Autodesk Fusion 360 part; units mm, degrees
note: some values were not read from the file. Chosen so that the rebuilt part matches the saved one: which face or edge a step refers to. Set by a fixed rule: which sketch regions a step uses.
(part 2 of 7)
  arc A150 (-15.4464, 34.8123) -> (-14.944, 34.6491) centre (-15.1024, 35.0164) ccw
  spline S149 degree 3 poles (-19.866, 37.3046) (-19.823, 35.7503) (-19.6037, 34.6096) (-19.3931, 33.8552) knots 0 0 0 0 1 1 1 1
  arc A151 (-20.7021, 31.9674) -> (-20.1803, 31.8848) centre (-20.3942, 32.2228) ccw
  spline S150 degree 3 poles (-10.2263, 37.6523) (-10.6107, 38.3346) (-11.2623, 39.2962) (-12.331, 40.4257) knots 0 0 0 0 1 1 1 1
  spline S151 degree 3 poles (-13.8582, 36.4722) (-13.808, 36.0399) (-13.7432, 35.732) (-13.6938, 35.5383) knots 0 0 0 0 1 1 1 1
  arc A152 (-8.2763, 36.8156) -> (-9.3397, 36.5603) centre (0, 0) ccw
  spline S152 degree 3 poles (-1.9094, 38.9695) (-1.9952, 38.5429) (-2.0288, 38.23) (-2.0416, 38.0306) knots 0 0 0 0 1 1 1 1
  spline S153 degree 3 poles (-20.7021, 31.9674) (-20.8297, 32.1213) (-21.0408, 32.3546) (-21.3609, 32.6493) knots 0 0 0 0 1 1 1 1
  arc A153 (-19.2479, 32.4562) -> (-20.1803, 31.8848) centre (0, 0) ccw
  spline S154 degree 3 poles (-7.9821, 38.191) (-8.0001, 37.7562) (-7.9843, 37.442) (-7.9658, 37.243) knots 0 0 0 0 1 1 1 1
  arc A154 (-9.8104, 36.8001) -> (-9.3397, 36.5603) centre (-9.4387, 36.9478) ccw
  arc A155 (-13.9336, 35.0676) -> (-14.944, 34.6491) centre (0, 0) ccw
  spline S155 degree 3 poles (-13.7857, 39.953) (-13.9863, 38.4112) (-13.9482, 37.2502) (-13.8582, 36.4722) knots 0 0 0 0 1 1 1 1
  arc A156 (-18.5031, 37.999) -> (-19.866, 37.3046) centre (0, 0) ccw
  arc A157 (-19.2479, 32.4562) -> (-19.0846, 32.9586) centre (-19.4519, 32.8002) ccw
  arc A158 (-24.0882, 29.0455) -> (-24.0055, 29.5673) centre (-24.3435, 29.3534) ccw
  spline S156 degree 3 poles (-25.4571, 33.7376) (-25.1715, 32.2092) (-24.7765, 31.1168) (-24.4505, 30.4047) knots 0 0 0 0 1 1 1 1
  arc A159 (-24.2197, 34.6367) -> (-25.4571, 33.7376) centre (0, 0) ccw
  arc A160 (-24.0882, 29.0455) -> (-24.9197, 28.3353) centre (0, 0) ccw
  spline S157 degree 3 poles (-15.9905, 35.5889) (-16.477, 36.2028) (-17.271, 37.0506) (-18.5031, 37.999) knots 0 0 0 0 1 1 1 1
  spline S158 degree 3 poles (-19.3931, 33.8552) (-19.2759, 33.4362) (-19.1638, 33.1422) (-19.0846, 32.9586) knots 0 0 0 0 1 1 1 1
  spline S159 degree 3 poles (-21.3609, 32.6493) (-21.9375, 33.1795) (-22.8543, 33.8927) (-24.2197, 34.6367) knots 0 0 0 0 1 1 1 1
extrude "Extrude1'" add sketch "sketch 26269" along normal blind 8 separate body makes body 2 in component "Spur Gear (40 teeth)"
sketch "Sketch1 (2)" plane through (0, 0, 0) normal (0, 1, 0) x (1, 0, 0) in component "Spur Gear (40 teeth)"
  circle A0 centre (0, 0) radius 40.25 construction
sketch "sketch 33723" plane through (0, 0, 0) normal (0, 1, 0) x (1, 0, 0)
  arc A0 (-65.084, 44.4151) -> (-65.9408, 43.1328) centre (0, 0) ccw
  arc A1 (-66.3817, 42.9661) -> (-65.9408, 43.1328) centre (-66.2755, 43.3518) ccw
  arc A2 (-65.084, 44.4151) -> (-65.0987, 44.8863) centre (-65.4144, 44.6406) ccw
  arc A3 (-66.0742, 48.9963) -> (-67.0163, 47.6996) centre (0, 0) ccw
  arc A4 (-61.3986, 49.3846) -> (-62.3533, 48.1735) centre (0, 0) ccw
  spline S0 degree 3 poles (-66.9941, 43.1264) (-66.7812, 43.0736) (-66.5772, 43.02) (-66.3817, 42.9661) knots 0 0 0 0 1 1 1 1
  spline S1 degree 3 poles (-65.0987, 44.8863) (-65.2233, 45.0463) (-65.3508, 45.2143) (-65.4811, 45.3907) knots 0 0 0 0 1 1 1 1
  arc A5 (-58.8431, 52.8215) -> (-58.3815, 52.9172) centre (-58.6778, 53.1858) ccw
  arc A6 (-57.3346, 54.0497) -> (-58.3815, 52.9172) centre (0, 0) ccw
  spline S2 degree 3 poles (-62.0263, 54.0294) (-61.0366, 53.717) (-60.1704, 53.3921) (-59.4228, 53.0756) knots 0 0 0 0 1 1 1 1
  spline S3 degree 3 poles (-63.4039, 48.2497) (-63.1959, 48.1804) (-62.9966, 48.111) (-62.806, 48.0419) knots 0 0 0 0 1 1 1 1
  arc A7 (-62.806, 48.0419) -> (-62.3533, 48.1735) centre (-62.6699, 48.418) ccw
  spline S4 degree 3 poles (-61.7179, 50.3883) (-62.1475, 51.0772) (-62.6039, 51.8819) (-63.0673, 52.8106) knots 0 0 0 0 1 1 1 1
  spline S5 degree 3 poles (-61.3763, 49.8555) (-61.4879, 50.0247) (-61.6019, 50.2023) (-61.7179, 50.3883) knots 0 0 0 0 1 1 1 1
  spline S6 degree 3 poles (-65.4811, 45.3907) (-65.9633, 46.0437) (-66.4815, 46.8101) (-67.0163, 47.6996) knots 0 0 0 0 1 1 1 1
  arc A8 (-57.3346, 54.0497) -> (-57.2755, 54.5174) centre (-57.6257, 54.324) ccw
  arc A9 (-61.3986, 49.3846) -> (-61.3763, 49.8555) centre (-61.7102, 49.6353) ccw
  spline S7 degree 3 poles (-66.0742, 48.9963) (-65.063, 48.7626) (-64.174, 48.5066) (-63.4039, 48.2497) knots 0 0 0 0 1 1 1 1
  arc A10 (-62.0263, 54.0294) -> (-63.0673, 52.8106) centre (0, 0) ccw
  spline S8 degree 3 poles (-52.8106, 63.0673) (-51.8819, 62.6039) (-51.0772, 62.1475) (-50.3883, 61.7179) knots 0 0 0 0 1 1 1 1
  spline S9 degree 3 poles (-59.4228, 53.0756) (-59.2209, 52.9901) (-59.0277, 52.9053) (-58.8431, 52.8215) knots 0 0 0 0 1 1 1 1
  spline S10 degree 3 poles (-57.2755, 54.5174) (-57.3735, 54.6948) (-57.4732, 54.8807) (-57.5742, 55.0753) knots 0 0 0 0 1 1 1 1
  arc A11 (-57.596, 58.7294) -> (-58.7294, 57.596) centre (0, 0) ccw
  spline S11 degree 3 poles (-57.5742, 55.0753) (-57.9484, 55.7958) (-58.3403, 56.6338) (-58.7294, 57.596) knots 0 0 0 0 1 1 1 1
  spline S12 degree 3 poles (-57.596, 58.7294) (-56.6338, 58.3403) (-55.7958, 57.9484) (-55.0753, 57.5742) knots 0 0 0 0 1 1 1 1
  spline S13 degree 3 poles (-55.0753, 57.5742) (-54.8807, 57.4732) (-54.6948, 57.3735) (-54.5174, 57.2755) knots 0 0 0 0 1 1 1 1
  arc A12 (-52.9172, 58.3815) -> (-52.8215, 58.8431) centre (-53.1858, 58.6778) ccw
  arc A13 (-54.5174, 57.2755) -> (-54.0497, 57.3346) centre (-54.324, 57.6257) ccw
  arc A14 (-52.9172, 58.3815) -> (-54.0497, 57.3346) centre (0, 0) ccw
  spline S14 degree 3 poles (-50.3883, 61.7179) (-50.2023, 61.6019) (-50.0247, 61.4879) (-49.8555, 61.3763) knots 0 0 0 0 1 1 1 1
  spline S15 degree 3 poles (-52.8215, 58.8431) (-52.9053, 59.0277) (-52.9901, 59.2209) (-53.0756, 59.4228) knots 0 0 0 0 1 1 1 1
  spline S16 degree 3 poles (-48.0419, 62.806) (-48.111, 62.9966) (-48.1804, 63.1959) (-48.2497, 63.4039) knots 0 0 0 0 1 1 1 1
  arc A15 (-48.1735, 62.3533) -> (-49.3846, 61.3986) centre (0, 0) ccw
  arc A16 (-52.8106, 63.0673) -> (-54.0294, 62.0263) centre (0, 0) ccw
  spline S17 degree 3 poles (-53.0756, 59.4228) (-53.3921, 60.1704) (-53.717, 61.0366) (-54.0294, 62.0263) knots 0 0 0 0 1 1 1 1
  arc A17 (-49.8555, 61.3763) -> (-49.3846, 61.3986) centre (-49.6353, 61.7102) ccw
  spline S18 degree 3 poles (-47.6996, 67.0163) (-46.8101, 66.4815) (-46.0437, 65.9633) (-45.3907, 65.4811) knots 0 0 0 0 1 1 1 1
  spline S19 degree 3 poles (-48.2497, 63.4039) (-48.5066, 64.174) (-48.7626, 65.063) (-48.9963, 66.0742) knots 0 0 0 0 1 1 1 1
  arc A18 (-48.1735, 62.3533) -> (-48.0419, 62.806) centre (-48.418, 62.6699) ccw
  spline S20 degree 3 poles (-45.3907, 65.4811) (-45.2143, 65.3508) (-45.0463, 65.2233) (-44.8863, 65.0987) knots 0 0 0 0 1 1 1 1
  arc A19 (-43.1328, 65.9408) -> (-44.4151, 65.084) centre (0, 0) ccw
  arc A20 (-43.1328, 65.9408) -> (-42.9661, 66.3817) centre (-43.3518, 66.2755) ccw
  spline S21 degree 3 poles (-42.9661, 66.3817) (-43.02, 66.5772) (-43.0736, 66.7812) (-43.1264, 66.9941) knots 0 0 0 0 1 1 1 1
  arc A21 (-44.8863, 65.0987) -> (-44.4151, 65.084) centre (-44.6406, 65.4144) ccw
  spline S22 degree 3 poles (-42.2945, 70.5522) (-41.4498, 69.9493) (-40.7264, 69.3726) (-40.1132, 68.8406) knots 0 0 0 0 1 1 1 1
  arc A22 (-39.6403, 68.4198) -> (-39.1718, 68.3681) centre (-39.3706, 68.7152) ccw
  arc A23 (-47.6996, 67.0163) -> (-48.9963, 66.0742) centre (0, 0) ccw
  arc A24 (-42.2945, 70.5522) -> (-43.6612, 69.7147) centre (0, 0) ccw
  spline S23 degree 3 poles (-40.1132, 68.8406) (-39.9475, 68.6969) (-39.79, 68.5565) (-39.6403, 68.4198) knots 0 0 0 0 1 1 1 1
  spline S24 degree 3 poles (-37.7371, 70.1712) (-37.8704, 70.972) (-37.9841, 71.8901) (-38.0568, 72.9254) knots 0 0 0 0 1 1 1 1
  spline S25 degree 3 poles (-37.6254, 69.5482) (-37.6638, 69.7473) (-37.7012, 69.9549) (-37.7371, 70.1712) knots 0 0 0 0 1 1 1 1
  spline S26 degree 3 poles (-43.1264, 66.9941) (-43.322, 67.7819) (-43.5075, 68.6883) (-43.6612, 69.7147) knots 0 0 0 0 1 1 1 1
  arc A25 (-37.8262, 69.1217) -> (-39.1718, 68.3681) centre (0, 0) ccw
  spline S27 degree 3 poles (-30.737, 76.2999) (-29.997, 75.5723) (-29.3727, 74.8895) (-28.8503, 74.2681) knots 0 0 0 0 1 1 1 1
  arc A26 (-34.15, 71.319) -> (-33.6869, 71.2307) centre (-33.8579, 71.5923) ccw
  arc A27 (-26.5475, 74.188) -> (-27.9944, 73.6542) centre (0, 0) ccw
  arc A28 (-26.5475, 74.188) -> (-26.2825, 74.5778) centre (-26.6822, 74.5646) ccw
  spline S28 degree 3 poles (-34.5883, 71.7756) (-34.4345, 71.6193) (-34.2885, 71.4671) (-34.15, 71.319) knots 0 0 0 0 1 1 1 1
  arc A29 (-32.2864, 71.8764) -> (-32.0528, 72.2858) centre (-32.4503, 72.2413) ccw
  arc A30 (-36.6287, 73.6531) -> (-38.0568, 72.9254) centre (0, 0) ccw
  spline S29 degree 3 poles (-32.0528, 72.2858) (-32.0754, 72.4873) (-32.0964, 72.6972) (-32.1152, 72.9157) knots 0 0 0 0 1 1 1 1
  arc A31 (-30.737, 76.2999) -> (-32.2178, 75.6865) centre (0, 0) ccw
  spline S30 degree 3 poles (-26.2825, 74.5778) (-26.2892, 74.7805) (-26.2937, 74.9914) (-26.2953, 75.2107) knots 0 0 0 0 1 1 1 1
  arc A32 (-32.2864, 71.8764) -> (-33.6869, 71.2307) centre (0, 0) ccw
  spline S31 degree 3 poles (-28.8503, 74.2681) (-28.7092, 74.1003) (-28.5755, 73.937) (-28.4491, 73.7785) knots 0 0 0 0 1 1 1 1
  arc A33 (-37.8262, 69.1217) -> (-37.6254, 69.5482) centre (-38.0182, 69.4726) ccw
  spline S32 degree 3 poles (-36.6287, 73.6531) (-35.8338, 72.9858) (-35.1579, 72.3541) (-34.5883, 71.7756) knots 0 0 0 0 1 1 1 1
  spline S33 degree 3 poles (-32.1152, 72.9157) (-32.1852, 73.7245) (-32.2266, 74.6487) (-32.2178, 75.6865) knots 0 0 0 0 1 1 1 1
  arc A34 (-28.4491, 73.7785) -> (-27.9944, 73.6542) centre (-28.1365, 74.0281) ccw
  spline S34 degree 3 poles (-26.2953, 75.2107) (-26.3016, 76.0225) (-26.2704, 76.9471) (-26.1802, 77.981) knots 0 0 0 0 1 1 1 1
  arc A35 (-24.6558, 78.4763) -> (-26.1802, 77.981) centre (0, 0) ccw
  arc A36 (-20.6449, 76.0422) -> (-22.1292, 75.6235) centre (0, 0) ccw
  arc A37 (-20.6449, 76.0422) -> (-20.3501, 76.41) centre (-20.7497, 76.4282) ccw
  spline S35 degree 3 poles (-24.6558, 78.4763) (-23.9752, 77.6928) (-23.4064, 76.9632) (-22.9343, 76.3027) knots 0 0 0 0 1 1 1 1
  spline S36 degree 3 poles (-22.9343, 76.3027) (-22.8068, 76.1243) (-22.6864, 75.9511) (-22.5728, 75.7832) knots 0 0 0 0 1 1 1 1
  arc A38 (-22.5728, 75.7832) -> (-22.1292, 75.6235) centre (-22.2416, 76.0074) ccw
  spline S37 degree 3 poles (-20.3133, 77.0419) (-20.2559, 77.8517) (-20.1522, 78.771) (-19.9812, 79.7947) knots 0 0 0 0 1 1 1 1
  arc A39 (-18.4227, 80.1689) -> (-19.9812, 79.7947) centre (0, 0) ccw
  arc A40 (-14.6151, 77.4275) -> (-14.2923, 77.7712) centre (-14.6893, 77.8206) ccw
  spline S38 degree 3 poles (-20.3501, 76.41) (-20.341, 76.6126) (-20.3288, 76.8232) (-20.3133, 77.0419) knots 0 0 0 0 1 1 1 1
  spline S39 degree 3 poles (-18.4227, 80.1689) (-17.8055, 79.3344) (-17.2958, 78.5624) (-16.877, 77.8669) knots 0 0 0 0 1 1 1 1
  spline S40 degree 3 poles (-14.2061, 78.3982) (-14.0853, 79.201) (-13.9098, 80.1093) (-13.659, 81.1164) knots 0 0 0 0 1 1 1 1
  arc A41 (-16.5573, 77.3206) -> (-16.1277, 77.1267) centre (-16.2095, 77.5182) ccw
  arc A42 (-14.6151, 77.4275) -> (-16.1277, 77.1267) centre (0, 0) ccw
  arc A43 (-12.0759, 81.3672) -> (-13.659, 81.1164) centre (0, 0) ccw
  spline S41 degree 3 poles (-14.2923, 77.7712) (-14.2673, 77.9723) (-14.2387, 78.1814) (-14.2061, 78.3982) knots 0 0 0 0 1 1 1 1
  spline S42 degree 3 poles (-16.877, 77.8669) (-16.7639, 77.6791) (-16.6574, 77.4969) (-16.5573, 77.3206) knots 0 0 0 0 1 1 1 1
  spline S43 degree 3 poles (-12.0759, 81.3672) (-11.5261, 80.4868) (-11.0785, 79.6772) (-10.7156, 78.951) knots 0 0 0 0 1 1 1 1
  arc A44 (-5.6547, 82.0638) -> (-7.2526, 81.938) centre (0, 0) ccw
  arc A45 (-10.4398, 78.3813) -> (-10.0267, 78.1543) centre (-10.0776, 78.551) ccw
  spline S44 degree 3 poles (-10.7156, 78.951) (-10.6176, 78.7549) (-10.5258, 78.5649) (-10.4398, 78.3813) knots 0 0 0 0 1 1 1 1
  arc A46 (-8.4951, 78.3355) -> (-10.0267, 78.1543) centre (0, 0) ccw
  arc A47 (-8.4951, 78.3355) -> (-8.1464, 78.6528) centre (-8.5383, 78.7332) ccw
  spline S45 degree 3 poles (-8.0112, 79.2711) (-7.8278, 80.0619) (-7.5816, 80.9537) (-7.2526, 81.938) knots 0 0 0 0 1 1 1 1
  spline S46 degree 3 poles (-8.1464, 78.6528) (-8.1057, 78.8514) (-8.0608, 79.0575) (-8.0112, 79.2711) knots 0 0 0 0 1 1 1 1
  arc A48 (-78.1543, 10.0267) -> (-78.3355, 8.4951) centre (0, 0) ccw
  arc A49 (-77.1267, 16.1277) -> (-77.3206, 16.5573) centre (-77.5182, 16.2095) ccw
  spline S47 degree 3 poles (-77.8669, 16.877) (-78.5624, 17.2958) (-79.3344, 17.8055) (-80.1689, 18.4227) knots 0 0 0 0 1 1 1 1
  arc A50 (-79.7947, 19.9812) -> (-80.1689, 18.4227) centre (0, 0) ccw
  spline S48 degree 3 poles (-81.1164, 13.659) (-80.1093, 13.9098) (-79.201, 14.0853) (-78.3982, 14.2061) knots 0 0 0 0 1 1 1 1
  spline S49 degree 3 poles (-78.3982, 14.2061) (-78.1814, 14.2387) (-77.9723, 14.2673) (-77.7712, 14.2923) knots 0 0 0 0 1 1 1 1
  arc A51 (-75.6235, 22.1292) -> (-76.0422, 20.6449) centre (0, 0) ccw
  arc A52 (-77.1267, 16.1277) -> (-77.4275, 14.6151) centre (0, 0) ccw
  arc A53 (-75.6235, 22.1292) -> (-75.7832, 22.5728) centre (-76.0074, 22.2416) ccw
  spline S50 degree 3 poles (-79.7947, 19.9812) (-78.771, 20.1522) (-77.8517, 20.2559) (-77.0419, 20.3133) knots 0 0 0 0 1 1 1 1
  spline S51 degree 3 poles (-77.0419, 20.3133) (-76.8232, 20.3288) (-76.6126, 20.341) (-76.41, 20.3501) knots 0 0 0 0 1 1 1 1
  arc A54 (-78.6528, 8.1464) -> (-78.3355, 8.4951) centre (-78.7332, 8.5383) ccw
  arc A55 (-78.1543, 10.0267) -> (-78.3813, 10.4398) centre (-78.551, 10.0776) ccw
  spline S52 degree 3 poles (-78.3813, 10.4398) (-78.5649, 10.5258) (-78.7549, 10.6176) (-78.951, 10.7156) knots 0 0 0 0 1 1 1 1
  spline S53 degree 3 poles (-79.2711, 8.0112) (-79.0575, 8.0608) (-78.8514, 8.1057) (-78.6528, 8.1464) knots 0 0 0 0 1 1 1 1
  arc A56 (-77.7712, 14.2923) -> (-77.4275, 14.6151) centre (-77.8206, 14.6893) ccw
  arc A57 (-81.1164, 13.659) -> (-81.3672, 12.0759) centre (0, 0) ccw
  spline S54 degree 3 poles (-78.951, 10.7156) (-79.6772, 11.0785) (-80.4868, 11.5261) (-81.3672, 12.0759) knots 0 0 0 0 1 1 1 1
  spline S55 degree 3 poles (-77.3206, 16.5573) (-77.4969, 16.6574) (-77.6791, 16.7639) (-77.8669, 16.877) knots 0 0 0 0 1 1 1 1
  spline S56 degree 3 poles (-77.981, 26.1802) (-76.9471, 26.2704) (-76.0225, 26.3016) (-75.2107, 26.2953) knots 0 0 0 0 1 1 1 1
  spline S57 degree 3 poles (-74.2681, 28.8503) (-74.8895, 29.3727) (-75.5723, 29.997) (-76.2999, 30.737) knots 0 0 0 0 1 1 1 1
  arc A58 (-75.6865, 32.2178) -> (-76.2999, 30.737) centre (0, 0) ccw
  arc A59 (-71.2307, 33.6869) -> (-71.8764, 32.2864) centre (0, 0) ccw
  spline S58 degree 3 poles (-75.6865, 32.2178) (-74.6487, 32.2266) (-73.7245, 32.1852) (-72.9157, 32.1152) knots 0 0 0 0 1 1 1 1
  spline S59 degree 3 poles (-73.7785, 28.4491) (-73.937, 28.5755) (-74.1003, 28.7092) (-74.2681, 28.8503) knots 0 0 0 0 1 1 1 1
  spline S60 degree 3 poles (-71.319, 34.15) (-71.4671, 34.2885) (-71.6193, 34.4345) (-71.7756, 34.5883) knots 0 0 0 0 1 1 1 1
  arc A60 (-76.41, 20.3501) -> (-76.0422, 20.6449) centre (-76.4282, 20.7497) ccw
  spline S61 degree 3 poles (-76.3027, 22.9343) (-76.9632, 23.4064) (-77.6928, 23.9752) (-78.4763, 24.6558) knots 0 0 0 0 1 1 1 1
  spline S62 degree 3 poles (-75.7832, 22.5728) (-75.9511, 22.6864) (-76.1243, 22.8068) (-76.3027, 22.9343) knots 0 0 0 0 1 1 1 1
  spline S63 degree 3 poles (-75.2107, 26.2953) (-74.9914, 26.2937) (-74.7805, 26.2892) (-74.5778, 26.2825) knots 0 0 0 0 1 1 1 1
  arc A61 (-77.981, 26.1802) -> (-78.4763, 24.6558) centre (0, 0) ccw
  arc A62 (-74.5778, 26.2825) -> (-74.188, 26.5475) centre (-74.5646, 26.6822) ccw
  arc A63 (-73.6542, 27.9944) -> (-73.7785, 28.4491) centre (-74.0281, 28.1365) ccw
  arc A64 (-73.6542, 27.9944) -> (-74.188, 26.5475) centre (0, 0) ccw
  spline S64 degree 3 poles (-68.8406, 40.1132) (-69.3726, 40.7264) (-69.9493, 41.4498) (-70.5522, 42.2945) knots 0 0 0 0 1 1 1 1
  spline S65 degree 3 poles (-69.7147, 43.6612) (-68.6883, 43.5075) (-67.7819, 43.322) (-66.9941, 43.1264) knots 0 0 0 0 1 1 1 1
  arc A65 (-71.2307, 33.6869) -> (-71.319, 34.15) centre (-71.5923, 33.8579) ccw
  arc A66 (-72.2858, 32.0528) -> (-71.8764, 32.2864) centre (-72.2413, 32.4503) ccw
  spline S66 degree 3 poles (-72.9254, 38.0568) (-71.8901, 37.9841) (-70.972, 37.8704) (-70.1712, 37.7371) knots 0 0 0 0 1 1 1 1
  spline S67 degree 3 poles (-71.7756, 34.5883) (-72.3541, 35.1579) (-72.9858, 35.8338) (-73.6531, 36.6287) knots 0 0 0 0 1 1 1 1
  arc A67 (-72.9254, 38.0568) -> (-73.6531, 36.6287) centre (0, 0) ccw
  spline S68 degree 3 poles (-68.4198, 39.6403) (-68.5565, 39.79) (-68.6969, 39.9475) (-68.8406, 40.1132) knots 0 0 0 0 1 1 1 1
  arc A68 (-69.5482, 37.6254) -> (-69.1217, 37.8262) centre (-69.4726, 38.0182) ccw
  spline S69 degree 3 poles (-70.1712, 37.7371) (-69.9549, 37.7012) (-69.7473, 37.6638) (-69.5482, 37.6254) knots 0 0 0 0 1 1 1 1
  spline S70 degree 3 poles (-72.9157, 32.1152) (-72.6972, 32.0964) (-72.4873, 32.0754) (-72.2858, 32.0528) knots 0 0 0 0 1 1 1 1
  arc A69 (-68.3681, 39.1718) -> (-68.4198, 39.6403) centre (-68.7152, 39.3706) ccw
  arc A70 (-68.3681, 39.1718) -> (-69.1217, 37.8262) centre (0, 0) ccw
  arc A71 (71.2307, -33.6869) -> (71.8764, -32.2864) centre (0, 0) ccw
  spline S71 degree 3 poles (72.9157, -32.1152) (72.6972, -32.0964) (72.4873, -32.0754) (72.2858, -32.0528) knots 0 0 0 0 1 1 1 1
  arc A72 (72.9254, -38.0568) -> (73.6531, -36.6287) centre (0, 0) ccw
  spline S72 degree 3 poles (71.319, -34.15) (71.4671, -34.2885) (71.6193, -34.4345) (71.7756, -34.5883) knots 0 0 0 0 1 1 1 1
  spline S73 degree 3 poles (72.9254, -38.0568) (71.8901, -37.9841) (70.972, -37.8704) (70.1712, -37.7371) knots 0 0 0 0 1 1 1 1
  spline S74 degree 3 poles (71.7756, -34.5883) (72.3541, -35.1579) (72.9858, -35.8338) (73.6531, -36.6287) knots 0 0 0 0 1 1 1 1
  spline S75 degree 3 poles (68.4198, -39.6403) (68.5565, -39.79) (68.6969, -39.9475) (68.8406, -40.1132) knots 0 0 0 0 1 1 1 1
  arc A73 (68.3681, -39.1718) -> (69.1217, -37.8262) centre (0, 0) ccw
  arc A74 (68.3681, -39.1718) -> (68.4198, -39.6403) centre (68.7152, -39.3706) ccw
  spline S76 degree 3 poles (75.6865, -32.2178) (74.6487, -32.2266) (73.7245, -32.1852) (72.9157, -32.1152) knots 0 0 0 0 1 1 1 1
  arc A75 (-69.7147, 43.6612) -> (-70.5522, 42.2945) centre (0, 0) ccw
  arc A76 (71.2307, -33.6869) -> (71.319, -34.15) centre (71.5923, -33.8579) ccw
  arc A77 (72.2858, -32.0528) -> (71.8764, -32.2864) centre (72.2413, -32.4503) ccw
  arc A78 (69.5482, -37.6254) -> (69.1217, -37.8262) centre (69.4726, -38.0182) ccw
  spline S77 degree 3 poles (70.1712, -37.7371) (69.9549, -37.7012) (69.7473, -37.6638) (69.5482, -37.6254) knots 0 0 0 0 1 1 1 1
  spline S78 degree 3 poles (68.8406, -40.1132) (69.3726, -40.7264) (69.9493, -41.4498) (70.5522, -42.2945) knots 0 0 0 0 1 1 1 1
  arc A79 (69.7147, -43.6612) -> (70.5522, -42.2945) centre (0, 0) ccw
  spline S79 degree 3 poles (69.7147, -43.6612) (68.6883, -43.5075) (67.7819, -43.322) (66.9941, -43.1264) knots 0 0 0 0 1 1 1 1
  arc A80 (66.0742, -48.9963) -> (67.0163, -47.6996) centre (0, 0) ccw
  arc A81 (65.084, -44.4151) -> (65.9408, -43.1328) centre (0, 0) ccw
  arc A82 (52.9172, -58.3815) -> (54.0497, -57.3346) centre (0, 0) ccw
  spline S80 degree 3 poles (61.7179, -50.3883) (62.1475, -51.0772) (62.6039, -51.8819) (63.0673, -52.8106) knots 0 0 0 0 1 1 1 1
  arc A83 (58.8431, -52.8215) -> (58.3815, -52.9172) centre (58.6778, -53.1858) ccw
  arc A84 (52.9172, -58.3815) -> (52.8215, -58.8431) centre (53.1858, -58.6778) ccw
  spline S81 degree 3 poles (52.8106, -63.0673) (51.8819, -62.6039) (51.0772, -62.1475) (50.3883, -61.7179) knots 0 0 0 0 1 1 1 1
  arc A85 (65.084, -44.4151) -> (65.0987, -44.8863) centre (65.4144, -44.6406) ccw
  arc A86 (61.3986, -49.3846) -> (62.3533, -48.1735) centre (0, 0) ccw
  arc A87 (61.3986, -49.3846) -> (61.3763, -49.8555) centre (61.7102, -49.6353) ccw
  spline S82 degree 3 poles (65.0987, -44.8863) (65.2233, -45.0463) (65.3508, -45.2143) (65.4811, -45.3907) knots 0 0 0 0 1 1 1 1
  spline S83 degree 3 poles (62.0263, -54.0294) (61.0366, -53.717) (60.1704, -53.3921) (59.4228, -53.0756) knots 0 0 0 0 1 1 1 1
  arc A88 (62.806, -48.0419) -> (62.3533, -48.1735) centre (62.6699, -48.418) ccw
  spline S84 degree 3 poles (57.5742, -55.0753) (57.9484, -55.7958) (58.3403, -56.6338) (58.7294, -57.596) knots 0 0 0 0 1 1 1 1
  arc A89 (52.8106, -63.0673) -> (54.0294, -62.0263) centre (0, 0) ccw
  spline S85 degree 3 poles (50.3883, -61.7179) (50.2023, -61.6019) (50.0247, -61.4879) (49.8555, -61.3763) knots 0 0 0 0 1 1 1 1
  arc A90 (57.596, -58.7294) -> (58.7294, -57.596) centre (0, 0) ccw
  spline S86 degree 3 poles (66.9941, -43.1264) (66.7812, -43.0736) (66.5772, -43.02) (66.3817, -42.9661) knots 0 0 0 0 1 1 1 1
  spline S87 degree 3 poles (65.4811, -45.3907) (65.9633, -46.0437) (66.4815, -46.8101) (67.0163, -47.6996) knots 0 0 0 0 1 1 1 1
  arc A91 (48.1735, -62.3533) -> (49.3846, -61.3986) centre (0, 0) ccw
  spline S88 degree 3 poles (57.596, -58.7294) (56.6338, -58.3403) (55.7958, -57.9484) (55.0753, -57.5742) knots 0 0 0 0 1 1 1 1
  spline S89 degree 3 poles (52.8215, -58.8431) (52.9053, -59.0277) (52.9901, -59.2209) (53.0756, -59.4228) knots 0 0 0 0 1 1 1 1
  spline S90 degree 3 poles (59.4228, -53.0756) (59.2209, -52.9901) (59.0277, -52.9053) (58.8431, -52.8215) knots 0 0 0 0 1 1 1 1
  spline S91 degree 3 poles (55.0753, -57.5742) (54.8807, -57.4732) (54.6948, -57.3735) (54.5174, -57.2755) knots 0 0 0 0 1 1 1 1
  spline S92 degree 3 poles (61.3763, -49.8555) (61.4879, -50.0247) (61.6019, -50.2023) (61.7179, -50.3883) knots 0 0 0 0 1 1 1 1
  spline S93 degree 3 poles (66.0742, -48.9963) (65.063, -48.7626) (64.174, -48.5066) (63.4039, -48.2497) knots 0 0 0 0 1 1 1 1
  spline S94 degree 3 poles (53.0756, -59.4228) (53.3921, -60.1704) (53.717, -61.0366) (54.0294, -62.0263) knots 0 0 0 0 1 1 1 1
  arc A92 (66.3817, -42.9661) -> (65.9408, -43.1328) centre (66.2755, -43.3518) ccw
  arc A93 (62.0263, -54.0294) -> (63.0673, -52.8106) centre (0, 0) ccw
  arc A94 (57.3346, -54.0497) -> (57.2755, -54.5174) centre (57.6257, -54.324) ccw
  spline S95 degree 3 poles (57.2755, -54.5174) (57.3735, -54.6948) (57.4732, -54.8807) (57.5742, -55.0753) knots 0 0 0 0 1 1 1 1
  arc A95 (54.5174, -57.2755) -> (54.0497, -57.3346) centre (54.324, -57.6257) ccw
  spline S96 degree 3 poles (63.4039, -48.2497) (63.1959, -48.1804) (62.9966, -48.111) (62.806, -48.0419) knots 0 0 0 0 1 1 1 1
  arc A96 (57.3346, -54.0497) -> (58.3815, -52.9172) centre (0, 0) ccw
  spline S97 degree 3 poles (48.0419, -62.806) (48.111, -62.9966) (48.1804, -63.1959) (48.2497, -63.4039) knots 0 0 0 0 1 1 1 1
  spline S98 degree 3 poles (48.2497, -63.4039) (48.5066, -64.174) (48.7626, -65.063) (48.9963, -66.0742) knots 0 0 0 0 1 1 1 1
  spline S99 degree 3 poles (47.6996, -67.0163) (46.8101, -66.4815) (46.0437, -65.9633) (45.3907, -65.4811) knots 0 0 0 0 1 1 1 1
  arc A97 (49.8555, -61.3763) -> (49.3846, -61.3986) centre (49.6353, -61.7102) ccw
  arc A98 (48.1735, -62.3533) -> (48.0419, -62.806) centre (48.418, -62.6699) ccw
  arc A99 (47.6996, -67.0163) -> (48.9963, -66.0742) centre (0, 0) ccw
  spline S100 degree 3 poles (43.1264, -66.9941) (43.322, -67.7819) (43.5075, -68.6883) (43.6612, -69.7147) knots 0 0 0 0 1 1 1 1
  arc A100 (42.2945, -70.5522) -> (43.6612, -69.7147) centre (0, 0) ccw
  spline S101 degree 3 poles (42.9661, -66.3817) (43.02, -66.5772) (43.0736, -66.7812) (43.1264, -66.9941) knots 0 0 0 0 1 1 1 1
  arc A101 (43.1328, -65.9408) -> (42.9661, -66.3817) centre (43.3518, -66.2755) ccw
  arc A102 (43.1328, -65.9408) -> (44.4151, -65.084) centre (0, 0) ccw
  spline S102 degree 3 poles (45.3907, -65.4811) (45.2143, -65.3508) (45.0463, -65.2233) (44.8863, -65.0987) knots 0 0 0 0 1 1 1 1
  arc A103 (37.8262, -69.1217) -> (37.6254, -69.5482) centre (38.0182, -69.4726) ccw
  arc A104 (39.6403, -68.4198) -> (39.1718, -68.3681) centre (39.3706, -68.7152) ccw
  arc A105 (37.8262, -69.1217) -> (39.1718, -68.3681) centre (0, 0) ccw
  spline S103 degree 3 poles (42.2945, -70.5522) (41.4498, -69.9493) (40.7264, -69.3726) (40.1132, -68.8406) knots 0 0 0 0 1 1 1 1
  arc A106 (36.6287, -73.6531) -> (38.0568, -72.9254) centre (0, 0) ccw
  spline S104 degree 3 poles (37.6254, -69.5482) (37.6638, -69.7473) (37.7012, -69.9549) (37.7371, -70.1712) knots 0 0 0 0 1 1 1 1
  arc A107 (44.8863, -65.0987) -> (44.4151, -65.084) centre (44.6406, -65.4144) ccw
  spline S105 degree 3 poles (37.7371, -70.1712) (37.8704, -70.972) (37.9841, -71.8901) (38.0568, -72.9254) knots 0 0 0 0 1 1 1 1
  spline S106 degree 3 poles (40.1132, -68.8406) (39.9475, -68.6969) (39.79, -68.5565) (39.6403, -68.4198) knots 0 0 0 0 1 1 1 1
  spline S107 degree 3 poles (36.6287, -73.6531) (35.8338, -72.9858) (35.1579, -72.3541) (34.5883, -71.7756) knots 0 0 0 0 1 1 1 1
  arc A108 (32.2864, -71.8764) -> (32.0528, -72.2858) centre (32.4503, -72.2413) ccw
  spline S108 degree 3 poles (32.0528, -72.2858) (32.0754, -72.4873) (32.0964, -72.6972) (32.1152, -72.9157) knots 0 0 0 0 1 1 1 1
  spline S109 degree 3 poles (34.5883, -71.7756) (34.4345, -71.6193) (34.2885, -71.4671) (34.15, -71.319) knots 0 0 0 0 1 1 1 1
  arc A109 (30.737, -76.2999) -> (32.2178, -75.6865) centre (0, 0) ccw
  spline S110 degree 3 poles (30.737, -76.2999) (29.997, -75.5723) (29.3727, -74.8895) (28.8503, -74.2681) knots 0 0 0 0 1 1 1 1
  arc A110 (34.15, -71.319) -> (33.6869, -71.2307) centre (33.8579, -71.5923) ccw
  arc A111 (32.2864, -71.8764) -> (33.6869, -71.2307) centre (0, 0) ccw
  spline S111 degree 3 poles (32.1152, -72.9157) (32.1852, -73.7245) (32.2266, -74.6487) (32.2178, -75.6865) knots 0 0 0 0 1 1 1 1
  spline S112 degree 3 poles (24.6558, -78.4763) (23.9752, -77.6928) (23.4064, -76.9632) (22.9343, -76.3027) knots 0 0 0 0 1 1 1 1
  arc A112 (22.5728, -75.7832) -> (22.1292, -75.6235) centre (22.2416, -76.0074) ccw
  arc A113 (20.6449, -76.0422) -> (22.1292, -75.6235) centre (0, 0) ccw
  spline S113 degree 3 poles (20.3501, -76.41) (20.341, -76.6126) (20.3288, -76.8232) (20.3133, -77.0419) knots 0 0 0 0 1 1 1 1
  spline S114 degree 3 poles (22.9343, -76.3027) (22.8068, -76.1243) (22.6864, -75.9511) (22.5728, -75.7832) knots 0 0 0 0 1 1 1 1
  spline S115 degree 3 poles (20.3133, -77.0419) (20.2559, -77.8517) (20.1522, -78.771) (19.9812, -79.7947) knots 0 0 0 0 1 1 1 1
  arc A114 (14.6151, -77.4275) -> (14.2923, -77.7712) centre (14.6893, -77.8206) ccw
  spline S116 degree 3 poles (28.8503, -74.2681) (28.7092, -74.1003) (28.5755, -73.937) (28.4491, -73.7785) knots 0 0 0 0 1 1 1 1
  spline S117 degree 3 poles (18.4227, -80.1689) (17.8055, -79.3344) (17.2958, -78.5624) (16.877, -77.8669) knots 0 0 0 0 1 1 1 1
  arc A115 (16.5573, -77.3206) -> (16.1277, -77.1267) centre (16.2095, -77.5182) ccw
  spline S118 degree 3 poles (26.2825, -74.5778) (26.2892, -74.7805) (26.2937, -74.9914) (26.2953, -75.2107) knots 0 0 0 0 1 1 1 1
  arc A116 (14.6151, -77.4275) -> (16.1277, -77.1267) centre (0, 0) ccw
  arc A117 (20.6449, -76.0422) -> (20.3501, -76.41) centre (20.7497, -76.4282) ccw
  spline S119 degree 3 poles (16.877, -77.8669) (16.7639, -77.6791) (16.6574, -77.4969) (16.5573, -77.3206) knots 0 0 0 0 1 1 1 1
  spline S120 degree 3 poles (26.2953, -75.2107) (26.3016, -76.0225) (26.2704, -76.9471) (26.1802, -77.981) knots 0 0 0 0 1 1 1 1
  arc A118 (18.4227, -80.1689) -> (19.9812, -79.7947) centre (0, 0) ccw
  spline S121 degree 3 poles (14.2923, -77.7712) (14.2673, -77.9723) (14.2387, -78.1814) (14.2061, -78.3982) knots 0 0 0 0 1 1 1 1
  arc A119 (26.5475, -74.188) -> (27.9944, -73.6542) centre (0, 0) ccw
  arc A120 (28.4491, -73.7785) -> (27.9944, -73.6542) centre (28.1365, -74.0281) ccw
  arc A121 (26.5475, -74.188) -> (26.2825, -74.5778) centre (26.6822, -74.5646) ccw
  arc A122 (24.6558, -78.4763) -> (26.1802, -77.981) centre (0, 0) ccw
  arc A123 (12.0759, -81.3672) -> (13.659, -81.1164) centre (0, 0) ccw
  spline S122 degree 3 poles (14.2061, -78.3982) (14.0853, -79.201) (13.9098, -80.1093) (13.659, -81.1164) knots 0 0 0 0 1 1 1 1
  arc A124 (10.4398, -78.3813) -> (10.0267, -78.1543) centre (10.0776, -78.551) ccw
  spline S123 degree 3 poles (10.7156, -78.951) (10.6176, -78.7549) (10.5258, -78.5649) (10.4398, -78.3813) knots 0 0 0 0 1 1 1 1
  arc A125 (8.4951, -78.3355) -> (10.0267, -78.1543) centre (0, 0) ccw
  spline S124 degree 3 poles (12.0759, -81.3672) (11.5261, -80.4868) (11.0785, -79.6772) (10.7156, -78.951) knots 0 0 0 0 1 1 1 1
  arc A126 (-10.0267, -78.1543) -> (-10.4398, -78.3813) centre (-10.0776, -78.551) ccw
  spline S125 degree 3 poles (4.4881, -79.5484) (4.4058, -79.3452) (4.3292, -79.1486) (4.2579, -78.9588) knots 0 0 0 0 1 1 1 1
  arc A127 (4.2579, -78.9588) -> (3.8638, -78.7) centre (3.8835, -79.0995) ccw
  spline S126 degree 3 poles (-4.2579, -78.9588) (-4.3292, -79.1486) (-4.4058, -79.3452) (-4.4881, -79.5484) knots 0 0 0 0 1 1 1 1
  arc A128 (-7.2526, -81.938) -> (-5.6547, -82.0638) centre (0, 0) ccw
  arc A129 (5.6547, -82.0638) -> (7.2526, -81.938) centre (0, 0) ccw
  arc A130 (2.3228, -78.7606) -> (1.9503, -79.0495) centre (2.3346, -79.1604) ccw
  spline S127 degree 3 poles (-8.0112, -79.2711) (-8.0608, -79.0575) (-8.1057, -78.8514) (-8.1464, -78.6528) knots 0 0 0 0 1 1 1 1
  spline S128 degree 3 poles (-10.4398, -78.3813) (-10.5258, -78.5649) (-10.6176, -78.7549) (-10.7156, -78.951) knots 0 0 0 0 1 1 1 1
  spline S129 degree 3 poles (-13.659, -81.1164) (-13.9098, -80.1093) (-14.0853, -79.201) (-14.2061, -78.3982) knots 0 0 0 0 1 1 1 1
  spline S130 degree 3 poles (76.3027, -22.9343) (76.9632, -23.4064) (77.6928, -23.9752) (78.4763, -24.6558) knots 0 0 0 0 1 1 1 1
  arc A131 (77.981, -26.1802) -> (78.4763, -24.6558) centre (0, 0) ccw
  spline S131 degree 3 poles (75.7832, -22.5728) (75.9511, -22.6864) (76.1243, -22.8068) (76.3027, -22.9343) knots 0 0 0 0 1 1 1 1
  arc A132 (73.6542, -27.9944) -> (73.7785, -28.4491) centre (74.0281, -28.1365) ccw
  spline S132 degree 3 poles (75.2107, -26.2953) (74.9914, -26.2937) (74.7805, -26.2892) (74.5778, -26.2825) knots 0 0 0 0 1 1 1 1
  spline S133 degree 3 poles (73.7785, -28.4491) (73.937, -28.5755) (74.1003, -28.7092) (74.2681, -28.8503) knots 0 0 0 0 1 1 1 1
  arc A133 (2.3228, -78.7606) -> (3.8638, -78.7) centre (0, 0) ccw
  spline S134 degree 3 poles (8.1464, -78.6528) (8.1057, -78.8514) (8.0608, -79.0575) (8.0112, -79.2711) knots 0 0 0 0 1 1 1 1
  arc A134 (8.4951, -78.3355) -> (8.1464, -78.6528) centre (8.5383, -78.7332) ccw
  spline S135 degree 3 poles (8.0112, -79.2711) (7.8278, -80.0619) (7.5816, -80.9537) (7.2526, -81.938) knots 0 0 0 0 1 1 1 1
  spline S136 degree 3 poles (1.9503, -79.0495) (1.8941, -79.2443) (1.8331, -79.4462) (1.767, -79.6553) knots 0 0 0 0 1 1 1 1
  arc A135 (-1.9503, -79.0495) -> (-2.3228, -78.7606) centre (-2.3346, -79.1604) ccw
  arc A136 (-8.1464, -78.6528) -> (-8.4951, -78.3355) centre (-8.5383, -78.7332) ccw
  spline S137 degree 3 poles (5.6547, -82.0638) (5.1757, -81.1431) (4.793, -80.3008) (4.4881, -79.5484) knots 0 0 0 0 1 1 1 1
  spline S138 degree 3 poles (1.767, -79.6553) (1.5221, -80.4293) (1.2067, -81.299) (0.8014, -82.2545) knots 0 0 0 0 1 1 1 1
  arc A137 (-3.8638, -78.7) -> (-2.3228, -78.7606) centre (0, 0) ccw
  spline S139 degree 3 poles (-7.2526, -81.938) (-7.5816, -80.9537) (-7.8278, -80.0619) (-8.0112, -79.2711) knots 0 0 0 0 1 1 1 1
  spline S140 degree 3 poles (-1.767, -79.6553) (-1.8331, -79.4462) (-1.8941, -79.2443) (-1.9503, -79.0495) knots 0 0 0 0 1 1 1 1
  arc A138 (-13.659, -81.1164) -> (-12.0759, -81.3672) centre (0, 0) ccw
  spline S141 degree 3 poles (-0.8014, -82.2545) (-1.2067, -81.299) (-1.5221, -80.4293) (-1.767, -79.6553) knots 0 0 0 0 1 1 1 1
  spline S142 degree 3 poles (-10.7156, -78.951) (-11.0785, -79.6772) (-11.5261, -80.4868) (-12.0759, -81.3672) knots 0 0 0 0 1 1 1 1
  arc A139 (-0.8014, -82.2545) -> (0.8014, -82.2545) centre (0, 0) ccw
  arc A140 (-14.2923, -77.7712) -> (-14.6151, -77.4275) centre (-14.6893, -77.8206) ccw
  arc A141 (-16.1277, -77.1267) -> (-14.6151, -77.4275) centre (0, 0) ccw
  spline S143 degree 3 poles (77.981, -26.1802) (76.9471, -26.2704) (76.0225, -26.3016) (75.2107, -26.2953) knots 0 0 0 0 1 1 1 1
  arc A142 (-10.0267, -78.1543) -> (-8.4951, -78.3355) centre (0, 0) ccw
  spline S144 degree 3 poles (-14.2061, -78.3982) (-14.2387, -78.1814) (-14.2673, -77.9723) (-14.2923, -77.7712) knots 0 0 0 0 1 1 1 1
  spline S145 degree 3 poles (-4.4881, -79.5484) (-4.793, -80.3008) (-5.1757, -81.1431) (-5.6547, -82.0638) knots 0 0 0 0 1 1 1 1
  arc A143 (-3.8638, -78.7) -> (-4.2579, -78.9588) centre (-3.8835, -79.0995) ccw
  spline S146 degree 3 poles (-45.3907, -65.4811) (-46.0437, -65.9633) (-46.8101, -66.4815) (-47.6996, -67.0163) knots 0 0 0 0 1 1 1 1
  spline S147 degree 3 poles (-34.15, -71.319) (-34.2885, -71.4671) (-34.4345, -71.6193) (-34.5883, -71.7756) knots 0 0 0 0 1 1 1 1
  arc A144 (-38.0568, -72.9254) -> (-36.6287, -73.6531) centre (0, 0) ccw
  spline S148 degree 3 poles (-48.2497, -63.4039) (-48.1804, -63.1959) (-48.111, -62.9966) (-48.0419, -62.806) knots 0 0 0 0 1 1 1 1
  spline S149 degree 3 poles (-53.0756, -59.4228) (-52.9901, -59.2209) (-52.9053, -59.0277) (-52.8215, -58.8431) knots 0 0 0 0 1 1 1 1
  arc A145 (-52.8215, -58.8431) -> (-52.9172, -58.3815) centre (-53.1858, -58.6778) ccw
  spline S150 degree 3 poles (-40.1132, -68.8406) (-40.7264, -69.3726) (-41.4498, -69.9493) (-42.2945, -70.5522) knots 0 0 0 0 1 1 1 1
  spline S151 degree 3 poles (74.2681, -28.8503) (74.8895, -29.3727) (75.5723, -29.997) (76.2999, -30.737) knots 0 0 0 0 1 1 1 1
  spline S152 degree 3 poles (-38.0568, -72.9254) (-37.9841, -71.8901) (-37.8704, -70.972) (-37.7371, -70.1712) knots 0 0 0 0 1 1 1 1
  arc A146 (74.5778, -26.2825) -> (74.188, -26.5475) centre (74.5646, -26.6822) ccw
  spline S153 degree 3 poles (-43.1264, -66.9941) (-43.0736, -66.7812) (-43.02, -66.5772) (-42.9661, -66.3817) knots 0 0 0 0 1 1 1 1
  arc A147 (-54.0497, -57.3346) -> (-54.5174, -57.2755) centre (-54.324, -57.6257) ccw
  arc A148 (-39.1718, -68.3681) -> (-39.6403, -68.4198) centre (-39.3706, -68.7152) ccw
  spline S154 degree 3 poles (-50.3883, -61.7179) (-51.0772, -62.1475) (-51.8819, -62.6039) (-52.8106, -63.0673) knots 0 0 0 0 1 1 1 1
  spline S155 degree 3 poles (-34.5883, -71.7756) (-35.1579, -72.3541) (-35.8338, -72.9858) (-36.6287, -73.6531) knots 0 0 0 0 1 1 1 1
  arc A149 (-44.4151, -65.084) -> (-44.8863, -65.0987) centre (-44.6406, -65.4144) ccw
  spline S156 degree 3 poles (-55.0753, -57.5742) (-55.7958, -57.9484) (-56.6338, -58.3403) (-57.596, -58.7294) knots 0 0 0 0 1 1 1 1
  arc A150 (-37.6254, -69.5482) -> (-37.8262, -69.1217) centre (-38.0182, -69.4726) ccw
  spline S157 degree 3 poles (-43.6612, -69.7147) (-43.5075, -68.6883) (-43.322, -67.7819) (-43.1264, -66.9941) knots 0 0 0 0 1 1 1 1
  spline S158 degree 3 poles (-39.6403, -68.4198) (-39.79, -68.5565) (-39.9475, -68.6969) (-40.1132, -68.8406) knots 0 0 0 0 1 1 1 1
  arc A151 (-44.4151, -65.084) -> (-43.1328, -65.9408) centre (0, 0) ccw
  arc A152 (-42.9661, -66.3817) -> (-43.1328, -65.9408) centre (-43.3518, -66.2755) ccw
  arc A153 (-48.9963, -66.0742) -> (-47.6996, -67.0163) centre (0, 0) ccw
  arc A154 (-48.0419, -62.806) -> (-48.1735, -62.3533) centre (-48.418, -62.6699) ccw
  spline S159 degree 3 poles (-48.9963, -66.0742) (-48.7626, -65.063) (-48.5066, -64.174) (-48.2497, -63.4039) knots 0 0 0 0 1 1 1 1
  arc A155 (-54.0294, -62.0263) -> (-52.8106, -63.0673) centre (0, 0) ccw
  spline S160 degree 3 poles (-54.5174, -57.2755) (-54.6948, -57.3735) (-54.8807, -57.4732) (-55.0753, -57.5742) knots 0 0 0 0 1 1 1 1
  arc A156 (-57.2755, -54.5174) -> (-57.3346, -54.0497) centre (-57.6257, -54.324) ccw
  spline S161 degree 3 poles (-58.7294, -57.596) (-58.3403, -56.6338) (-57.9484, -55.7958) (-57.5742, -55.0753) knots 0 0 0 0 1 1 1 1
  arc A157 (-49.3846, -61.3986) -> (-49.8555, -61.3763) centre (-49.6353, -61.7102) ccw
  arc A158 (-49.3846, -61.3986) -> (-48.1735, -62.3533) centre (0, 0) ccw
  spline S162 degree 3 poles (-49.8555, -61.3763) (-50.0247, -61.4879) (-50.2023, -61.6019) (-50.3883, -61.7179) knots 0 0 0 0 1 1 1 1
  arc A159 (75.6865, -32.2178) -> (76.2999, -30.737) centre (0, 0) ccw
  arc A160 (73.6542, -27.9944) -> (74.188, -26.5475) centre (0, 0) ccw
  arc A161 (-43.6612, -69.7147) -> (-42.2945, -70.5522) centre (0, 0) ccw
  arc A162 (-39.1718, -68.3681) -> (-37.8262, -69.1217) centre (0, 0) ccw
  spline S163 degree 3 poles (-37.7371, -70.1712) (-37.7012, -69.9549) (-37.6638, -69.7473) (-37.6254, -69.5482) knots 0 0 0 0 1 1 1 1
  arc A163 (-54.0497, -57.3346) -> (-52.9172, -58.3815) centre (0, 0) ccw
  spline S164 degree 3 poles (-54.0294, -62.0263) (-53.717, -61.0366) (-53.3921, -60.1704) (-53.0756, -59.4228) knots 0 0 0 0 1 1 1 1
  arc A164 (-58.7294, -57.596) -> (-57.596, -58.7294) centre (0, 0) ccw
  arc A165 (-58.3815, -52.9172) -> (-57.3346, -54.0497) centre (0, 0) ccw
  spline S165 degree 3 poles (-57.5742, -55.0753) (-57.4732, -54.8807) (-57.3735, -54.6948) (-57.2755, -54.5174) knots 0 0 0 0 1 1 1 1
  spline S166 degree 3 poles (-44.8863, -65.0987) (-45.0463, -65.2233) (-45.2143, -65.3508) (-45.3907, -65.4811) knots 0 0 0 0 1 1 1 1
  spline S167 degree 3 poles (-61.7179, -50.3883) (-61.6019, -50.2023) (-61.4879, -50.0247) (-61.3763, -49.8555) knots 0 0 0 0 1 1 1 1
  arc A166 (-62.3533, -48.1735) -> (-61.3986, -49.3846) centre (0, 0) ccw
  arc A167 (-69.1217, -37.8262) -> (-69.5482, -37.6254) centre (-69.4726, -38.0182) ccw
  spline S168 degree 3 poles (-67.0163, -47.6996) (-66.4815, -46.8101) (-65.9633, -46.0437) (-65.4811, -45.3907) knots 0 0 0 0 1 1 1 1
  spline S169 degree 3 poles (-63.4039, -48.2497) (-64.174, -48.5066) (-65.063, -48.7626) (-66.0742, -48.9963) knots 0 0 0 0 1 1 1 1
  spline S170 degree 3 poles (-66.3817, -42.9661) (-66.5772, -43.02) (-66.7812, -43.0736) (-66.9941, -43.1264) knots 0 0 0 0 1 1 1 1
  spline S171 degree 3 poles (-70.5522, -42.2945) (-69.9493, -41.4498) (-69.3726, -40.7264) (-68.8406, -40.1132) knots 0 0 0 0 1 1 1 1
  arc A168 (-73.6531, -36.6287) -> (-72.9254, -38.0568) centre (0, 0) ccw
  arc A169 (-68.4198, -39.6403) -> (-68.3681, -39.1718) centre (-68.7152, -39.3706) ccw
  arc A170 (-65.0987, -44.8863) -> (-65.084, -44.4151) centre (-65.4144, -44.6406) ccw
  arc A171 (-70.5522, -42.2945) -> (-69.7147, -43.6612) centre (0, 0) ccw
  arc A172 (-69.1217, -37.8262) -> (-68.3681, -39.1718) centre (0, 0) ccw
  spline S172 degree 3 poles (-59.4228, -53.0756) (-60.1704, -53.3921) (-61.0366, -53.717) (-62.0263, -54.0294) knots 0 0 0 0 1 1 1 1
  arc A173 (-61.3763, -49.8555) -> (-61.3986, -49.3846) centre (-61.7102, -49.6353) ccw
  spline S173 degree 3 poles (-58.8431, -52.8215) (-59.0277, -52.9053) (-59.2209, -52.9901) (-59.4228, -53.0756) knots 0 0 0 0 1 1 1 1
  arc A174 (-63.0673, -52.8106) -> (-62.0263, -54.0294) centre (0, 0) ccw
  arc A175 (-62.3533, -48.1735) -> (-62.806, -48.0419) centre (-62.6699, -48.418) ccw
  arc A176 (-67.0163, -47.6996) -> (-66.0742, -48.9963) centre (0, 0) ccw
  spline S174 degree 3 poles (-63.0673, -52.8106) (-62.6039, -51.8819) (-62.1475, -51.0772) (-61.7179, -50.3883) knots 0 0 0 0 1 1 1 1
  spline S175 degree 3 poles (-62.806, -48.0419) (-62.9966, -48.111) (-63.1959, -48.1804) (-63.4039, -48.2497) knots 0 0 0 0 1 1 1 1
  arc A177 (-65.9408, -43.1328) -> (-65.084, -44.4151) centre (0, 0) ccw
  spline S176 degree 3 poles (-65.4811, -45.3907) (-65.3508, -45.2143) (-65.2233, -45.0463) (-65.0987, -44.8863) knots 0 0 0 0 1 1 1 1
  spline S177 degree 3 poles (-66.9941, -43.1264) (-67.7819, -43.322) (-68.6883, -43.5075) (-69.7147, -43.6612) knots 0 0 0 0 1 1 1 1
  arc A178 (-65.9408, -43.1328) -> (-66.3817, -42.9661) centre (-66.2755, -43.3518) ccw
  spline S178 degree 3 poles (-68.8406, -40.1132) (-68.6969, -39.9475) (-68.5565, -39.79) (-68.4198, -39.6403) knots 0 0 0 0 1 1 1 1
  arc A179 (-58.3815, -52.9172) -> (-58.8431, -52.8215) centre (-58.6778, -53.1858) ccw
  spline S179 degree 3 poles (-78.4763, -24.6558) (-77.6928, -23.9752) (-76.9632, -23.4064) (-76.3027, -22.9343) knots 0 0 0 0 1 1 1 1
  spline S180 degree 3 poles (-74.5778, -26.2825) (-74.7805, -26.2892) (-74.9914, -26.2937) (-75.2107, -26.2953) knots 0 0 0 0 1 1 1 1
  arc A180 (-76.0422, -20.6449) -> (-76.41, -20.3501) centre (-76.4282, -20.7497) ccw
  spline S181 degree 3 poles (-76.3027, -22.9343) (-76.1243, -22.8068) (-75.9511, -22.6864) (-75.7832, -22.5728) knots 0 0 0 0 1 1 1 1
  arc A181 (-74.188, -26.5475) -> (-74.5778, -26.2825) centre (-74.5646, -26.6822) ccw
  spline S182 degree 3 poles (-76.41, -20.3501) (-76.6126, -20.341) (-76.8232, -20.3288) (-77.0419, -20.3133) knots 0 0 0 0 1 1 1 1
  arc A182 (-80.1689, -18.4227) -> (-79.7947, -19.9812) centre (0, 0) ccw
  spline S183 degree 3 poles (-80.1689, -18.4227) (-79.3344, -17.8055) (-78.5624, -17.2958) (-77.8669, -16.877) knots 0 0 0 0 1 1 1 1
  spline S184 degree 3 poles (-77.8669, -16.877) (-77.6791, -16.7639) (-77.4969, -16.6574) (-77.3206, -16.5573) knots 0 0 0 0 1 1 1 1
  arc A183 (-78.4763, -24.6558) -> (-77.981, -26.1802) centre (0, 0) ccw
  spline S185 degree 3 poles (-71.7756, -34.5883) (-71.6193, -34.4345) (-71.4671, -34.2885) (-71.319, -34.15) knots 0 0 0 0 1 1 1 1
  arc A184 (-73.7785, -28.4491) -> (-73.6542, -27.9944) centre (-74.0281, -28.1365) ccw
  arc A185 (-71.8764, -32.2864) -> (-72.2858, -32.0528) centre (-72.2413, -32.4503) ccw
  spline S186 degree 3 poles (-72.9157, -32.1152) (-73.7245, -32.1852) (-74.6487, -32.2266) (-75.6865, -32.2178) knots 0 0 0 0 1 1 1 1
  spline S187 degree 3 poles (-75.2107, -26.2953) (-76.0225, -26.3016) (-76.9471, -26.2704) (-77.981, -26.1802) knots 0 0 0 0 1 1 1 1
  arc A186 (-76.0422, -20.6449) -> (-75.6235, -22.1292) centre (0, 0) ccw
  spline S188 degree 3 poles (-72.2858, -32.0528) (-72.4873, -32.0754) (-72.6972, -32.0964) (-72.9157, -32.1152) knots 0 0 0 0 1 1 1 1
  arc A187 (-71.319, -34.15) -> (-71.2307, -33.6869) centre (-71.5923, -33.8579) ccw
  arc A188 (-76.2999, -30.737) -> (-75.6865, -32.2178) centre (0, 0) ccw
  spline S189 degree 3 poles (-70.1712, -37.7371) (-70.972, -37.8704) (-71.8901, -37.9841) (-72.9254, -38.0568) knots 0 0 0 0 1 1 1 1
  spline S190 degree 3 poles (-74.2681, -28.8503) (-74.1003, -28.7092) (-73.937, -28.5755) (-73.7785, -28.4491) knots 0 0 0 0 1 1 1 1
  arc A189 (-74.188, -26.5475) -> (-73.6542, -27.9944) centre (0, 0) ccw
  spline S191 degree 3 poles (-69.5482, -37.6254) (-69.7473, -37.6638) (-69.9549, -37.7012) (-70.1712, -37.7371) knots 0 0 0 0 1 1 1 1
  arc A190 (-71.8764, -32.2864) -> (-71.2307, -33.6869) centre (0, 0) ccw
  spline S192 degree 3 poles (-76.2999, -30.737) (-75.5723, -29.997) (-74.8895, -29.3727) (-74.2681, -28.8503) knots 0 0 0 0 1 1 1 1
  arc A191 (-75.7832, -22.5728) -> (-75.6235, -22.1292) centre (-76.0074, -22.2416) ccw
  spline S193 degree 3 poles (-73.6531, -36.6287) (-72.9858, -35.8338) (-72.3541, -35.1579) (-71.7756, -34.5883) knots 0 0 0 0 1 1 1 1
  spline S194 degree 3 poles (-81.3672, -12.0759) (-80.4868, -11.5261) (-79.6772, -11.0785) (-78.951, -10.7156) knots 0 0 0 0 1 1 1 1
  spline S195 degree 3 poles (-78.6528, -8.1464) (-78.8514, -8.1057) (-79.0575, -8.0608) (-79.2711, -8.0112) knots 0 0 0 0 1 1 1 1
  arc A192 (-77.4275, -14.6151) -> (-77.1267, -16.1277) centre (0, 0) ccw
  arc A193 (-77.3206, -16.5573) -> (-77.1267, -16.1277) centre (-77.5182, -16.2095) ccw
  spline S196 degree 3 poles (-77.7712, -14.2923) (-77.9723, -14.2673) (-78.1814, -14.2387) (-78.3982, -14.2061) knots 0 0 0 0 1 1 1 1
  arc A194 (-78.3355, -8.4951) -> (-78.1543, -10.0267) centre (0, 0) ccw
  spline S197 degree 3 poles (-79.2711, -8.0112) (-80.0619, -7.8278) (-80.9537, -7.5816) (-81.938, -7.2526) knots 0 0 0 0 1 1 1 1
  arc A195 (-78.3355, -8.4951) -> (-78.6528, -8.1464) centre (-78.7332, -8.5383) ccw
  arc A196 (-82.0638, -5.6547) -> (-81.938, -7.2526) centre (0, 0) ccw
  spline S198 degree 3 poles (-78.951, -10.7156) (-78.7549, -10.6176) (-78.5649, -10.5258) (-78.3813, -10.4398) knots 0 0 0 0 1 1 1 1
  arc A197 (-78.9588, -4.2579) -> (-78.7, -3.8638) centre (-79.0995, -3.8835) ccw
  arc A198 (-78.7606, -2.3228) -> (-78.7, -3.8638) centre (0, 0) ccw
  arc A199 (-78.7606, -2.3228) -> (-79.0495, -1.9503) centre (-79.1604, -2.3346) ccw
  spline S199 degree 3 poles (-77.0419, -20.3133) (-77.8517, -20.2559) (-78.771, -20.1522) (-79.7947, -19.9812) knots 0 0 0 0 1 1 1 1
  spline S200 degree 3 poles (-78.3982, -14.2061) (-79.201, -14.0853) (-80.1093, -13.9098) (-81.1164, -13.659) knots 0 0 0 0 1 1 1 1
  arc A200 (-81.3672, -12.0759) -> (-81.1164, -13.659) centre (0, 0) ccw
  arc A201 (-77.4275, -14.6151) -> (-77.7712, -14.2923) centre (-77.8206, -14.6893) ccw
  arc A202 (-78.3813, -10.4398) -> (-78.1543, -10.0267) centre (-78.551, -10.0776) ccw
  spline S201 degree 3 poles (-82.0638, -5.6547) (-81.1431, -5.1757) (-80.3008, -4.793) (-79.5484, -4.4881) knots 0 0 0 0 1 1 1 1
  spline S202 degree 3 poles (-79.6553, -1.767) (-80.4293, -1.5221) (-81.299, -1.2067) (-82.2545, -0.8014) knots 0 0 0 0 1 1 1 1
  spline S203 degree 3 poles (-79.0495, -1.9503) (-79.2443, -1.8941) (-79.4462, -1.8331) (-79.6553, -1.767) knots 0 0 0 0 1 1 1 1
  spline S204 degree 3 poles (-79.5484, -4.4881) (-79.3452, -4.4058) (-79.1486, -4.3292) (-78.9588, -4.2579) knots 0 0 0 0 1 1 1 1
  arc A203 (-82.2545, 0.8014) -> (-82.2545, -0.8014) centre (0, 0) ccw
  spline S205 degree 3 poles (-78.9588, 4.2579) (-79.1486, 4.3292) (-79.3452, 4.4058) (-79.5484, 4.4881) knots 0 0 0 0 1 1 1 1
  arc A204 (-79.0495, 1.9503) -> (-78.7606, 2.3228) centre (-79.1604, 2.3346) ccw
  arc A205 (-78.7, 3.8638) -> (-78.7606, 2.3228) centre (0, 0) ccw
  spline S206 degree 3 poles (-82.2545, 0.8014) (-81.299, 1.2067) (-80.4293, 1.5221) (-79.6553, 1.767) knots 0 0 0 0 1 1 1 1
  arc A206 (-78.7, 3.8638) -> (-78.9588, 4.2579) centre (-79.0995, 3.8835) ccw
  spline S207 degree 3 poles (-32.1152, -72.9157) (-32.0964, -72.6972) (-32.0754, -72.4873) (-32.0528, -72.2858) knots 0 0 0 0 1 1 1 1
  arc A207 (-32.0528, -72.2858) -> (-32.2864, -71.8764) centre (-32.4503, -72.2413) ccw
  arc A208 (-16.1277, -77.1267) -> (-16.5573, -77.3206) centre (-16.2095, -77.5182) ccw
  spline S208 degree 3 poles (-16.877, -77.8669) (-17.2958, -78.5624) (-17.8055, -79.3344) (-18.4227, -80.1689) knots 0 0 0 0 1 1 1 1
  arc A209 (-26.2825, -74.5778) -> (-26.5475, -74.188) centre (-26.6822, -74.5646) ccw
  arc A210 (-33.6869, -71.2307) -> (-32.2864, -71.8764) centre (0, 0) ccw
  spline S209 degree 3 poles (-1.767, 79.6553) (-1.5221, 80.4293) (-1.2067, 81.299) (-0.8014, 82.2545) knots 0 0 0 0 1 1 1 1
  spline S210 degree 3 poles (-26.1802, -77.981) (-26.2704, -76.9471) (-26.3016, -76.0225) (-26.2953, -75.2107) knots 0 0 0 0 1 1 1 1
  arc A211 (-32.2178, -75.6865) -> (-30.737, -76.2999) centre (0, 0) ccw
  arc A212 (0.8014, 82.2545) -> (-0.8014, 82.2545) centre (0, 0) ccw
  arc A213 (-22.1292, -75.6235) -> (-22.5728, -75.7832) centre (-22.2416, -76.0074) ccw
  arc A214 (-26.1802, -77.981) -> (-24.6558, -78.4763) centre (0, 0) ccw
  spline S211 degree 3 poles (-16.5573, -77.3206) (-16.6574, -77.4969) (-16.7639, -77.6791) (-16.877, -77.8669) knots 0 0 0 0 1 1 1 1
  spline S212 degree 3 poles (-19.9812, -79.7947) (-20.1522, -78.771) (-20.2559, -77.8517) (-20.3133, -77.0419) knots 0 0 0 0 1 1 1 1
  arc A215 (-27.9944, -73.6542) -> (-28.4491, -73.7785) centre (-28.1365, -74.0281) ccw
  spline S213 degree 3 poles (-79.6553, 1.767) (-79.4462, 1.8331) (-79.2443, 1.8941) (-79.0495, 1.9503) knots 0 0 0 0 1 1 1 1
  spline S214 degree 3 poles (-20.3133, -77.0419) (-20.3288, -76.8232) (-20.341, -76.6126) (-20.3501, -76.41) knots 0 0 0 0 1 1 1 1
  spline S215 degree 3 poles (-26.2953, -75.2107) (-26.2937, -74.9914) (-26.2892, -74.7805) (-26.2825, -74.5778) knots 0 0 0 0 1 1 1 1
  arc A216 (-20.3501, -76.41) -> (-20.6449, -76.0422) centre (-20.7497, -76.4282) ccw
  arc A217 (-22.1292, -75.6235) -> (-20.6449, -76.0422) centre (0, 0) ccw
  spline S216 degree 3 poles (-22.9343, -76.3027) (-23.4064, -76.9632) (-23.9752, -77.6928) (-24.6558, -78.4763) knots 0 0 0 0 1 1 1 1
  arc A218 (-81.938, 7.2526) -> (-82.0638, 5.6547) centre (0, 0) ccw
  spline S217 degree 3 poles (-22.5728, -75.7832) (-22.6864, -75.9511) (-22.8068, -76.1243) (-22.9343, -76.3027) knots 0 0 0 0 1 1 1 1
  spline S218 degree 3 poles (-28.8503, -74.2681) (-29.3727, -74.8895) (-29.997, -75.5723) (-30.737, -76.2999) knots 0 0 0 0 1 1 1 1
  spline S219 degree 3 poles (-32.2178, -75.6865) (-32.2266, -74.6487) (-32.1852, -73.7245) (-32.1152, -72.9157) knots 0 0 0 0 1 1 1 1
  arc A219 (-33.6869, -71.2307) -> (-34.15, -71.319) centre (-33.8579, -71.5923) ccw
  arc A220 (-19.9812, -79.7947) -> (-18.4227, -80.1689) centre (0, 0) ccw
  spline S220 degree 3 poles (-81.938, 7.2526) (-80.9537, 7.5816) (-80.0619, 7.8278) (-79.2711, 8.0112) knots 0 0 0 0 1 1 1 1
  spline S221 degree 3 poles (-79.5484, 4.4881) (-80.3008, 4.793) (-81.1431, 5.1757) (-82.0638, 5.6547) knots 0 0 0 0 1 1 1 1
  arc A221 (-27.9944, -73.6542) -> (-26.5475, -74.188) centre (0, 0) ccw
  spline S222 degree 3 poles (-28.4491, -73.7785) (-28.5755, -73.937) (-28.7092, -74.1003) (-28.8503, -74.2681) knots 0 0 0 0 1 1 1 1
  arc A222 (3.8638, 78.7) -> (4.2579, 78.9588) centre (3.8835, 79.0995) ccw
  spline S223 degree 3 poles (4.4881, 79.5484) (4.793, 80.3008) (5.1757, 81.1431) (5.6547, 82.0638) knots 0 0 0 0 1 1 1 1
  spline S224 degree 3 poles (7.2526, 81.938) (7.5816, 80.9537) (7.8278, 80.0619) (8.0112, 79.2711) knots 0 0 0 0 1 1 1 1
  arc A223 (10.0267, 78.1543) -> (8.4951, 78.3355) centre (0, 0) ccw
  arc A224 (8.1464, 78.6528) -> (8.4951, 78.3355) centre (8.5383, 78.7332) ccw
  arc A225 (10.0267, 78.1543) -> (10.4398, 78.3813) centre (10.0776, 78.551) ccw
  arc A226 (3.8638, 78.7) -> (2.3228, 78.7606) centre (0, 0) ccw